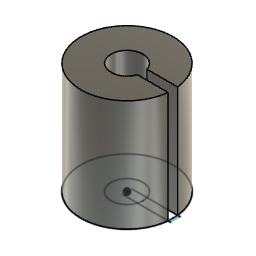
Adapter_Lenker v4 (Autodesk Fusion 360 design; units mm, degrees)
Autodesk Fusion 360 part; units mm, degrees
sketch "Skizze1" plane through (0, 0, 0) normal (0, 0, 1) x (1, 0, 0)
  circle A0 centre (0, 0) radius 14.5
  circle A1 centre (0, 0) radius 5
  line L0 (0, 1.5) -> (15.1231, 1.5)
  line L1 (15.1231, 1.5) -> (15.1231, -1.5)
  line L2 (15.1231, -1.5) -> (0, -1.5)
  line L3 (0, -1.5) -> (0, 1.5)
  dimension "d1" = 29
  dimension "d2" = 10
  dimension "d5" = 3
  dimension "d6" = 1.5
  constraint coincident A0.centre A1.centre
  constraint horizontal L0
  constraint vertical L1
  constraint horizontal L2
  constraint vertical L3
  measures "d1" diameter of A0
  measures "d2" diameter of A1
  measures "d5" distance of L0.start L2.end
  measures "d6" distance of A0.centre L0
extrude "Extrusion1" add sketch "Skizze1" along normal blind 35 contours A0 A1 L0 L2 picked at (-11.3068, 0)
equation "d1 = 25.9 mm + 3.1 mm"
equation "d6 = d5 / 2"
